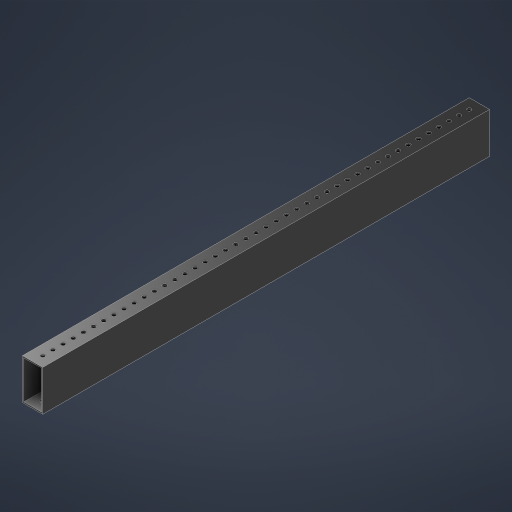
# Autodesk Inventor part: 6993, 22 in
Saved by Autodesk Inventor 2023 (Build 270158000, 158)
## iProperties
RuleStatus: InUse
Created: 2021-12-25
Part Number: 6993, 22 in
Material: Aluminum 6061
Document SubType Name: Modeling
Density: 2.7 g/cm^3
Appearance: Glossy - Black
AfterDocNew0: Configure
Autodesk Inventor part; units mm, degrees
ref_plane "YZ Plane" through (0, 0, 0) normal (1, 0, 0) x (0, 1, 0)
ref_plane "XZ Plane" through (0, 0, 0) normal (0, 1, 0) x (-1, 0, 0)
ref_plane "XY Plane" through (0, 0, 0) normal (0, 0, 1) x (1, 0, 0)
sketch "Sketch1" plane through (0, 0, 0) normal (0, 0, 1) x (1, 0, 0)
  line L0 (-12.7, -25.4) -> (12.7, -25.4)
  line L1 (12.7, -25.4) -> (12.7, 25.4)
  line L2 (12.7, 25.4) -> (-12.7, 25.4)
  line L3 (-12.7, 25.4) -> (-12.7, -25.4)
  line L4 (-12.7, -25.4) -> (12.7, 25.4) construction
  line L5 (12.7, -25.4) -> (-12.7, 25.4) construction
  line L6 (-11.1125, -23.8125) -> (11.1125, -23.8125)
  line L7 (11.1125, -23.8125) -> (11.1125, 23.8125)
  line L8 (11.1125, 23.8125) -> (-11.1125, 23.8125)
  line L9 (-11.1125, 23.8125) -> (-11.1125, -23.8125)
  point P0 (0, 0)
  dimension "d0" = 25.4
  dimension "d1" = 50.8
  dimension "d2" = 1.5875
  constraints: 20 end point, 4 parallel, 2 midpoint, 2 perpendicular, 1 horizontal, 3 other
  measures "d0" distance of L2.end L1.end
  measures "d1" distance of L1.end L0.end
  measures "d2" distance between parallel lines of L3 L9
extrude "BaseTube" add sketch "Sketch1" along normal mid plane 558.8
sketch "TopPoint" plane through (-12.7, 25.4, 279.4) normal (0, 1, 0) x (1, 0, 0)
  line L0 (25.4, 0) -> (0, 0) projected
  line L1 (0, 558.8) -> (0, 0) projected
  point P0 (12.7, 12.7)
  dimension "TLE_" = 12.7
  dimension "TWE_" = 12.7
  measures "TLE_" distance from line of L0 point (12.7, 12.7)
  measures "TWE_" distance from line of L1 point (12.7, 12.7)
sketch "SidePoint" plane through (12.7, -25.4, 279.4) normal (1, 0, 0) x (0, 0, -1)
  line L0 (0, 0) -> (0, 50.8) projected
  line L1 (558.8, 50.8) -> (0, 50.8) projected
  point P0 (12.7, 38.1)
  dimension "SLE_" = 12.7
  dimension "SWE_" = 12.7
  measures "SLE_" distance from line of point (12.7, 38.1) L0
  measures "SWE_" distance from line of point (12.7, 38.1) L1
hole "TopHole" at (0, 25.4, 266.7) direction (0, -1, 0) diameter 4.9784 end through all
hole "SideHole" [suppressed]
pattern_linear "TopPattern" count 22 spacing 12.7 along (0, 0, -1) of "TopHole"
pattern_linear "SidePattern" [suppressed]
mirror "TopMirror" about plane through (0, 0, 0) normal (0, 0, 1) of "TopHole", "TopPattern"
mirror "SideMirror" [suppressed]
sketch "Sketch4" plane through (-12.7, 25.4, 279.4) normal (0, 1, 0) x (1, 0, 0)
  line L0 (25.4, 558.8) -> (25.4, 0) projected
  line L1 (25.4, 0) -> (0, 0) projected
  line L2 (0, 558.8) -> (25.4, 558.8) projected
  line L3 (0, 558.8) -> (0, 0) projected
  line L4 (0, 0) -> (25.4, 25.4)
  line L5 (0, 558.8) -> (25.4, 533.4)
  dimension "d36" = 25.4
  constraints: 4 end point, 2 point on line, 1 perpendicular
  measures "d36" distance from line of L1 L4.end
extrude "CornerCut" [suppressed]
sketch "Sketch5" plane through (12.7, -25.4, 279.4) normal (1, 0, 0) x (0, 0, -1)
  circle A0 centre (31.75, 25.4) radius 14.2875
  line L0 (0, 0) -> (0, 50.8) projected
  point P0 (0, 25.4)
  dimension "d39" = 28.575
  dimension "d40" = 31.75
  constraints: 1 centre point, 1 horizontal alignment, 1 midpoint
  measures "d39" diameter of A0
  measures "d40" distance from line of A0.centre L0
extrude "FrontBearingHole" [suppressed]
sketch "Sketch6" plane through (12.7, -25.4, 279.4) normal (1, 0, 0) x (0, 0, -1)
  circle A0 centre (527.05, 25.4) radius 14.2875
  line L0 (558.8, 50.8) -> (558.8, 0) projected
  point P0 (558.8, 25.4)
  dimension "d43" = 28.575
  dimension "d44" = 31.75
  constraints: 1 centre point, 1 horizontal alignment, 1 midpoint
  measures "d43" diameter of A0
  measures "d44" distance from line of L0 A0.centre
extrude "BackBearingHole" [suppressed]
sketch "Drivetrain" plane through (0, -25.4, 254) normal (1, 0, 0) x (0, 0, -1)
  circle A0 centre (-46.0312, 25.4) radius 14.2875
  circle A1 centre (153.9875, 23.8125) radius 14.2875
  line L0 (533.4, 50.8) -> (-25.4, 50.8) construction
  line L1 (533.4, 0) -> (-25.4, 0) construction
  arc A2 (-45.8868, 43.5908) -> (-46.1756, 7.2092) centre (-46.0312, 25.4) ccw construction
  arc A3 (153.8431, 5.6217) -> (154.1319, 42.0033) centre (153.9875, 23.8125) ccw construction
  line L2 (-45.8868, 43.5908) -> (154.1319, 42.0033) construction
  line L3 (153.8431, 5.6217) -> (-46.1756, 7.2092) construction
  circle A4 centre (-46.0312, 25.4) radius 50.8 construction
  circle A5 centre (153.9875, 23.8125) radius 50.8 construction
  circle A6 centre (354.0125, 23.8125) radius 50.8 construction
  circle A7 centre (554.0312, 25.4) radius 50.8 construction
  line L4 (254, 50.8) -> (254, 0) construction
  line L5 (153.9875, 23.8125) -> (354.0125, 23.8125) construction
  line L6 (153.9875, 5.6211) -> (354.0125, 5.6211) construction
  line L7 (354.0125, 42.0039) -> (153.9875, 42.0039) construction
  arc A8 (153.9875, 42.0039) -> (153.9875, 5.6211) centre (153.9875, 23.8125) ccw construction
  arc A9 (354.0125, 5.6211) -> (354.0125, 42.0039) centre (354.0125, 23.8125) ccw construction
  circle A10 centre (-69.8437, 25.4) radius 2.4892
  circle A11 centre (130.175, 23.8125) radius 2.4892
  circle A12 centre (-62.8692, 8.562) radius 2.4892
  circle A13 centre (-46.0312, 1.5875) radius 2.4892 construction
  circle A14 centre (-29.1932, 8.562) radius 2.4892
  circle A15 centre (-22.2187, 25.4) radius 2.4892
  circle A16 centre (-29.1932, 42.238) radius 2.4892
  circle A17 centre (-46.0312, 49.2125) radius 2.4892 construction
  circle A18 centre (-62.8692, 42.238) radius 2.4892
  circle A19 centre (137.1495, 6.9745) radius 2.4892
  circle A20 centre (153.9875, 0) radius 2.4892 construction
  circle A21 centre (170.8255, 6.9745) radius 2.4892
  circle A22 centre (177.8, 23.8125) radius 2.4892
  circle A23 centre (170.8255, 40.6505) radius 2.4892
  circle A24 centre (153.9875, 47.625) radius 2.4892 construction
  circle A25 centre (137.1495, 40.6505) radius 2.4892
  circle A26 centre (-7.9312, 26.9875) radius 2.4892
  circle A27 centre (-7.9312, 26.9875) radius 4.7625
  circle A28 centre (192.0875, 26.9875) radius 2.4892
  circle A29 centre (192.0875, 26.9875) radius 4.7625
  circle A30 centre (296.8436, 23.8125) radius 2.4892
  circle A31 centre (411.1436, 23.8125) radius 2.4892
  circle A32 centre (296.8436, 23.8125) radius 4.7625
  circle A33 centre (411.1436, 23.8125) radius 4.7625
  line L8 (533.4, 50.8) -> (-25.4, 50.8) projected
  line L9 (260.35, 50.8) -> (260.35, 0) construction
  line L10 (-25.4, 50.8) -> (-25.4, 0) projected
  circle A34 centre (321.7831, -7114.6072) radius 1.0724
  circle A35 centre (321.7831, -7114.6072) radius 5.5468
  circle A36 centre (330.1811, 23.8125) radius 4.7625
  circle A37 centre (330.1811, 23.8125) radius 2.4892
  circle A38 centre (377.8061, 23.8125) radius 2.4892
  circle A39 centre (377.8061, 23.8125) radius 4.7625
  point P0 (254, 23.8125)
  point P1 (353.9936, 23.8125)
  point P2 (254, 25.4)
  dimension "d6" = 4.9784
  dimension "d47" = 28.575
  dimension "d52" = 25.4
  dimension "d64" = 26.9875
  dimension "d68" = 36.3828
  dimension "d69" = 57.15
  dimension "d70" = 200.025
  dimension "d71" = 57.15
  dimension "DTOuter" = 200.025
  dimension "d74" = 101.6
  dimension "d186" = 38.1
  dimension "d189" = 38.1
  dimension "d190" = 23.8125
  dimension "d306" = 57.15
  dimension "d307" = 200.025
  dimension "d308" = 57.15
  dimension "d310" = 4.9784
  dimension "d313" = 360
  dimension "d317" = 360
  dimension "d319" = 47.625
  dimension "d320" = 47.625
  dimension "d321" = 4.9784
  dimension "d322" = 9.525
  dimension "d331" = 4.9784
  dimension "d334" = 360
  dimension "d336" = 114.3
  dimension "GB_Height" = 26.9875
  dimension "GB_Front_Bearing_Height" = 1.5875
  dimension "d340" = 9.525
  dimension "d345" = 6.35
  dimension "DTInner" = 106.3625
  dimension "GB_Front_Bearing_Dist" = 379.3936
  dimension "d349" = -20.6312
  dimension "d350" = 47.625
  dimension "d351" = 33.3375
  dimension "d352" = 33.3375
  constraints: 40 centre point, 16 end point, 14 equal radius, 13 coincident, 8 horizontal alignment, 8 point on circle, 8 tangent, 3 midpoint, 2 parallel, 2 point on line, 2 symmetric about line, 1 horizontal, 1 perpendicular, 39 other
  measures "d47" diameter of A0
  measures "d52" distance from line of A0.centre L0
  measures "d64" distance from line of A1.centre L0
  measures "d68" diameter of A2
  measures "d70" distance of L3.start L3.end
  measures "DTOuter" distance of L2.start L2.end
  measures "d74" diameter of A4
  measures "d186" horizontal distance of A0.centre point (-7.931, 26.988)
  measures "d189" horizontal distance of point (192.087, 26.988) A1.centre
  measures "d190" distance from line of L0 point (-7.931, 26.988)
  measures "d307" distance of L6.start L6.end
  measures "d310" diameter of A10
  measures "d319" distance of A10.centre A15.centre
  measures "d320" distance of A22.centre A11.centre
  measures "d321" diameter of A26
  measures "d322" diameter of A27
  measures "d331" diameter of A30
  measures "d336" distance of A30.centre A31.centre
  measures "GB_Height" distance from line of point (353.994, 23.812) L0
  measures "GB_Front_Bearing_Height" vertical distance of A0.centre point (353.994, 23.812)
  measures "d340" diameter of A32
  measures "d345" distance between parallel lines of L9 L4
  measures "DTInner" distance from line of A1.centre L9
  measures "GB_Front_Bearing_Dist" horizontal distance of L0.end point (353.994, 23.812)
  measures "d349" distance from line of A0.centre L10
  measures "d350" distance of A39.centre A36.centre
  measures "d351" distance of A33.centre A38.centre
  measures "d352" distance of A30.centre A36.centre
extrude "Bearings" [suppressed]
extrude "BearingBlocks" [suppressed]
extrude "InsideCams" [suppressed]
extrude "OutsideCams" [suppressed]
mirror "DTMirror" [suppressed]
extrude "InsideGB" [suppressed]
extrude "OutsideGB" [suppressed]
feature "FrontGBCamDelete" [suppressed]
feature "FrontMidGBCamDelete" [suppressed]
feature "BackMidGBCamDelete" [suppressed]
feature "BackGBCamDelete" [suppressed]
equation "\"d0\" = Width"
equation "\"d1\" = Height"
equation "\"d2\" = Wall"
equation "\"d3\" = Length"
equation "\"d6\" = HoleSize"
equation "\"Height\" = 50.8"
equation "\"Width\" = 25.4"
equation "\"Wall\" = 1.5875"
equation "\"Length\" = 558.8"
equation "\"Top_Lengthwise_Space\" = 12.7"
equation "\"Top_Widthwise_Space\" = 12.7"
equation "\"Top_Lengthwise_Edge\" = 12.7"
equation "\"Top_Widthwise_Edge\" = 12.7"
equation "\"Side_Lengthwise_Edge\" = 12.7"
equation "\"Side_Widthwise_Edge\" = 12.7"
equation "\"Side_Lengthwise_Space\" = 12.7"
equation "\"Side_Widthwise_Space\" = 12.7"
equation "\"DT_Outer_Default\" = 200.025"
equation "\"DT_Inner_Default\" = 200.025"
equation "\"HoleSize\" = 4.9784"
body "Solid1"
